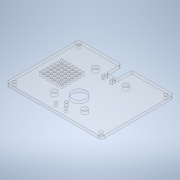
# Autodesk Inventor part: x_axis_plate_top_b
Saved by Autodesk Inventor 2022 (Build 260153000, 153)
## iProperties
Created: 2021-04-16
Part Number: x_axis_plate_top_b
Material: PET Plastic
Document SubType Name: Modeling
Designer: Fabijan_Sven
Density: 1.541 g/cm^3
Appearance: Polycarbonate - Clear
Mass: 163.421 g
Surface Area: 475.203 cm^2
Volume: 106.049 cm^3
Author: Fabijan_Sven
Autodesk Inventor part; units mm, degrees
ref_plane "YZ Plane" through (0, 0, 0) normal (1, 0, 0) x (0, 1, 0)
ref_plane "XZ Plane" through (0, 0, 0) normal (0, 1, 0) x (-1, 0, 0)
ref_plane "XY Plane" through (0, 0, 0) normal (0, 0, 1) x (1, 0, 0)
sketch "Sketch1" plane through (0, 0, 0) normal (0, 1, 0) x (-1, 0, 0)
  line L0 (81, 62) -> (-81, 62)
  line L1 (-81, 62) -> (-81, -62)
  line L2 (-81, -62) -> (81, -62)
  line L3 (81, -62) -> (81, 62)
  point P0 (0, 0)
  dimension "d127" = 162
  dimension "d128" = 81
  dimension "d129" = 124
  dimension "d130" = 62
  constraints: 8 end point, 2 parallel, 1 horizontal, 1 perpendicular
  measures "d127" distance between parallel lines of L1 L3
  measures "d128" distance from line of L1 point (0, 0)
  measures "d129" distance between parallel lines of L2 L0
  measures "d130" distance from line of point (0, 0) L0
extrude "Extrusion1" add sketch "Sketch1" along normal blind 5
fillet "Fillet1" radius 5 4 edges at (81, 2.5, 62) (-81, 2.5, 62) (-81, 2.5, -62) (81, 2.5, -62)
sketch "Sketch3" plane through (0, 5, 0) normal (0, 1, 0) x (1, 0, 0)
  circle A0 centre (74, -55) radius 3
  circle A1 centre (-74, -55) radius 3
  circle A2 centre (-74, 55) radius 3
  circle A3 centre (74, 55) radius 3
  line L0 (-81, 57) -> (-81, -57) projected
  line L1 (-76, -62) -> (76, -62) projected
  line L2 (81, -57) -> (81, 57) projected
  line L3 (76, 62) -> (-76, 62) projected
  point P0 (0, 0)
  dimension "d144" = 7
  dimension "d145" = 7
  dimension "d146" = 7
  dimension "d147" = 7
  dimension "d148" = 7
  dimension "d149" = 7
  dimension "d150" = 7
  dimension "d151" = 7
  dimension "d152" = 6
  constraints: 4 centre point, 3 equal radius
  measures "d144" distance from line of L0 A1.centre
  measures "d145" distance from line of L1 A1.centre
  measures "d146" distance from line of L1 A0.centre
  measures "d147" distance from line of L2 A0.centre
  measures "d148" distance from line of L2 A3.centre
  measures "d149" distance from line of L3 A3.centre
  measures "d150" distance from line of L3 A2.centre
  measures "d151" distance from line of L0 A2.centre
  measures "d152" diameter of A0
hole "Hole1" at (74, 5, 55) at (-74, 5, 55) at (74, 5, -55) at (-74, 5, -55) direction (0, -1, 0) diameter 6 end through all
sketch "Sketch4" plane through (0, 5, 0) normal (0, 1, 0) x (1, 0, 0)
  circle A0 centre (26.1863, -35) radius 5
  circle A1 centre (-26.1863, -35) radius 5
  circle A2 centre (0, 10.5) radius 5
  circle A3 centre (26.1863, 35) radius 5
  circle A4 centre (-26.1863, 35) radius 5
  point P0 (0, 0)
  dimension "d156" = 52.3726
  dimension "d157" = 70
  dimension "d158" = 24.5
  dimension "d159" = 26.1863
  dimension "d160" = 10
  dimension "d161" = 26.1863
  dimension "d162" = 35
  constraints: 5 centre point, 4 equal radius, 2 horizontal alignment, 2 vertical alignment
  measures "d156" distance of A1.centre A0.centre
  measures "d157" distance of A4.centre A1.centre
  measures "d158" vertical distance of A3.centre A2.centre
  measures "d159" horizontal distance of A2.centre A4.centre
  measures "d160" diameter of A1
  measures "d161" horizontal distance of point (0, 0) A1.centre
  measures "d162" vertical distance of point (0, 0) A1.centre
hole "Hole2" at (-26.1863, 5, 35) at (26.1863, 5, 35) at (26.1863, 5, -35) at (-26.1863, 5, -35) direction (0, -1, 0) diameter 10 end through all
sketch "Sketch5" plane through (0, 0, 0) normal (0, -1, 0) x (1, 0, 0)
  circle A0 centre (0, 18.5) radius 12
  line L0 (-76, 62) -> (76, 62) projected
  line L1 (-81, -57) -> (-81, 57) projected
  point P0 (0, 0)
  dimension "d33" = 24
  dimension "d131" = 43.5
  dimension "d132" = 81
  constraints: 1 centre point
  measures "d33" diameter of A0
  measures "d131" distance from line of L0 A0.centre
  measures "d132" distance from line of A0.centre L1
extrude "Extrusion3" cut sketch "Sketch5" against normal blind 10
sketch "Sketch7" plane through (0, 5, 0) normal (0, 1, 0) x (1, 0, 0)
  line L0 (9, 72) -> (-9, 72)
  line L1 (-9, 72) -> (-9, 37)
  line L2 (-9, 37) -> (9, 37)
  line L3 (9, 37) -> (9, 72)
  line L4 (76, 62) -> (-76, 62) projected
  point P0 (0, 0)
  point P1 (9, 62)
  point P2 (-9, 62)
  dimension "d133" = 18
  dimension "d134" = 35
  dimension "d136" = 10
  dimension "d137" = 9
  constraints: 8 end point, 2 parallel, 1 horizontal, 1 perpendicular
  measures "d133" distance between parallel lines of L3 L1
  measures "d134" distance between parallel lines of L0 L2
  measures "d136" distance between parallel lines of L4 L0
  measures "d137" distance from line of point (0, 0) L1
extrude "Extrusion5" cut sketch "Sketch7" against normal through all contours L3 L2 L1 L4
sketch "Sketch9" plane through (0, 5, 0) normal (0, 1, 0) x (1, 0, 0)
  circle A0 centre (-8.5, -49.5) radius 2.5
  circle A1 centre (8.5, -49.5) radius 2.5
  line L0 (-76, -62) -> (76, -62) projected
  line L1 (81, -57) -> (81, 57) projected
  line L2 (-81, 57) -> (-81, -57) projected
  dimension "d51" = 5
  dimension "d53" = 5
  dimension "d138" = 12.5
  dimension "d139" = 72.5
  dimension "d140" = 12.5
  dimension "d141" = 72.5
  constraints: 2 centre point
  measures "d51" diameter of A1
  measures "d53" diameter of A0
  measures "d138" distance from line of L0 A1.centre
  measures "d139" distance from line of L1 A1.centre
  measures "d140" distance from line of L0 A0.centre
  measures "d141" distance from line of L2 A0.centre
hole "Hole4" at (-8.5, 5, 49.5) at (8.5, 5, 49.5) direction (0, -1, 0) diameter 5 end through all
sketch "Sketch10" plane through (0, 5, 0) normal (0, 1, 0) x (1, 0, 0)
  circle A0 centre (0, -40) radius 3
  line L0 (-76, -62) -> (76, -62) projected
  line L1 (81, -57) -> (81, 57) projected
  dimension "d64" = 6
  dimension "d142" = 22
  dimension "d143" = 81
  constraints: 1 centre point
  measures "d64" diameter of A0
  measures "d142" distance from line of L0 A0.centre
  measures "d143" distance from line of L1 A0.centre
hole "Hole5" at (0, 5, 40) direction (0, -1, 0) diameter 6 depth 20 tip angle 118
sketch "Sketch13" plane through (0, 5, 0) normal (0, 1, 0) x (1, 0, 0)
  line L0 (9.2, 34) -> (5, 34)
  line L1 (5, 34) -> (5, 28.8)
  line L2 (5, 28.8) -> (9.2, 28.8)
  line L3 (9.2, 28.8) -> (9.2, 34)
  line L4 (-5, 34) -> (-9.2, 34)
  line L5 (-9.2, 34) -> (-9.2, 28.8)
  line L6 (-9.2, 28.8) -> (-5, 28.8)
  line L7 (-5, 28.8) -> (-5, 34)
  line L8 (-71, 37) -> (-91, 37) construction
  line L9 (9, 113) -> (9, 92) construction
  line L10 (9, 62) -> (9, 37) projected
  line L11 (9, 37) -> (-9, 37) projected
  point P0 (0, 0)
  dimension "d101" = 3
  dimension "d102" = 5.2
  dimension "d103" = 4.2
  dimension "d104" = 4.2
  dimension "d105" = 18.4
  dimension "d106" = 0.2
  dimension "d163" = 0
  dimension "d164" = 0
  constraints: 20 end point, 4 parallel, 2 horizontal, 2 perpendicular, 2 point on line
  measures "d101" distance between parallel lines of L0 L8
  measures "d102" distance between parallel lines of L0 L2
  measures "d103" distance between parallel lines of L1 L3
  measures "d104" distance between parallel lines of L7 L5
  measures "d105" distance between parallel lines of L3 L5
  measures "d106" distance between parallel lines of L9 L3
  measures "d163" distance between parallel lines of L10 L9
  measures "d164" distance between parallel lines of L11 L8
extrude "Extrusion7" cut sketch "Sketch13" against normal up to surface (5 mm away)
sketch "Sketch14" plane through (0.0871, 5, 4.1003) normal (0, 1, 0) x (1, 0, 0)
  circle A0 centre (-66.0871, 22.1003) radius 2
  line L0 (-95.5598, 66.1003) -> (-160.5598, 66.1003) construction
  line L1 (-81.0871, 110.2374) -> (-81.0871, -19.7626) construction
  circle A1 centre (-66.0871, 16.1003) radius 2
  circle A2 centre (-66.0871, 10.1003) radius 2
  circle A3 centre (-66.0871, 4.1003) radius 2
  circle A4 centre (-66.0871, -1.8997) radius 2
  circle A5 centre (-66.0871, -7.8997) radius 2
  circle A6 centre (-66.0871, -13.8997) radius 2
  circle A7 centre (-60.0871, 22.1003) radius 2
  circle A8 centre (-60.0871, 16.1003) radius 2
  circle A9 centre (-60.0871, 10.1003) radius 2
  circle A10 centre (-60.0871, 4.1003) radius 2
  circle A11 centre (-60.0871, -1.8997) radius 2
  circle A12 centre (-60.0871, -7.8997) radius 2
  circle A13 centre (-60.0871, -13.8997) radius 2
  circle A14 centre (-54.0871, 22.1003) radius 2
  circle A15 centre (-54.0871, 16.1003) radius 2
  circle A16 centre (-54.0871, 10.1003) radius 2
  circle A17 centre (-54.0871, 4.1003) radius 2
  circle A18 centre (-54.0871, -1.8997) radius 2
  circle A19 centre (-54.0871, -7.8997) radius 2
  circle A20 centre (-54.0871, -13.8997) radius 2
  circle A21 centre (-48.0871, 22.1003) radius 2
  circle A22 centre (-48.0871, 16.1003) radius 2
  circle A23 centre (-48.0871, 10.1003) radius 2
  circle A24 centre (-48.0871, 4.1003) radius 2
  circle A25 centre (-48.0871, -1.8997) radius 2
  circle A26 centre (-48.0871, -7.8997) radius 2
  circle A27 centre (-48.0871, -13.8997) radius 2
  circle A28 centre (-42.0871, 22.1003) radius 2
  circle A29 centre (-42.0871, 16.1003) radius 2
  circle A30 centre (-42.0871, 10.1003) radius 2
  circle A31 centre (-42.0871, 4.1003) radius 2
  circle A32 centre (-42.0871, -1.8997) radius 2
  circle A33 centre (-42.0871, -7.8997) radius 2
  circle A34 centre (-42.0871, -13.8997) radius 2
  circle A35 centre (-36.0871, 22.1003) radius 2
  circle A36 centre (-36.0871, 16.1003) radius 2
  circle A37 centre (-36.0871, 10.1003) radius 2
  circle A38 centre (-36.0871, 4.1003) radius 2
  circle A39 centre (-36.0871, -1.8997) radius 2
  circle A40 centre (-36.0871, -7.8997) radius 2
  circle A41 centre (-36.0871, -13.8997) radius 2
  circle A42 centre (-30.0871, 22.1003) radius 2
  circle A43 centre (-30.0871, 16.1003) radius 2
  circle A44 centre (-30.0871, 10.1003) radius 2
  circle A45 centre (-30.0871, 4.1003) radius 2
  circle A46 centre (-30.0871, -1.8997) radius 2
  circle A47 centre (-30.0871, -7.8997) radius 2
  circle A48 centre (-30.0871, -13.8997) radius 2
  line L2 (-9.0871, 66.1003) -> (-76.0871, 66.1003) projected
  line L3 (-81.0871, 61.1003) -> (-81.0871, -52.8997) projected
  point P0 (0, 0)
  dimension "d117" = 44
  dimension "d116" = 15
  dimension "d115" = 4
  dimension "d110" = 6
  dimension "d109" = 6
  dimension "d165" = 0
  dimension "d166" = 0
  constraints: 49 centre point, 4 end point, 1 horizontal, 1 vertical, 96 other
  measures "d117" distance from line of L0 A0.centre
  measures "d116" distance from line of L1 A0.centre
  measures "d115" diameter of A0
  measures "d110" distance of A0.centre A1.centre
  measures "d109" distance of A0.centre A7.centre
  measures "d165" distance between parallel lines of L2 L0
  measures "d166" distance between parallel lines of L3 L1
extrude "Extrusion8" cut sketch "Sketch14" against normal through all
fillet "Fillet4" radius 2 4 edges at (-9, 2.5, -62) (-9, 2.5, -37) (9, 2.5, -37) (9, 2.5, -62)
equation "\"d161\" = 0.5 * d156"
equation "\"d162\" = 0.5 * d157"
equation "\"d54\" = d53"
equation "\"d68\" = d64"
body "Solid1"
